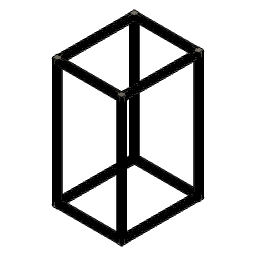
assembly (Autodesk Fusion 360 design; units mm, degrees)
Autodesk Fusion 360 part; units mm, degrees
sketch "Sketch1" plane through (0, 0, 0) normal (0, 0, 1) x (1, 0, 0) in component "2020-angle-connector"
  line L0 (10, 10) -> (-10, 10)
  line L1 (-10, 10) -> (-10, -10)
  line L2 (-10, -10) -> (10, -10)
  line L3 (10, -10) -> (10, 10)
  line L4 (10, 10) -> (-10, -10) construction
  line L5 (-10, 10) -> (10, -10) construction
  dimension "d1" = 20
  dimension "d2" = 20
  constraint horizontal L0
  constraint perpendicular L0 L1
  constraint parallel L0 L2
  constraint parallel L1 L3
  constraint coincident L4 origin
  constraint coincident L5 origin
  measures "d1" distance of L1.end L2.end
  measures "d2" distance of L0.end L1.end
extrude "Extrude1" add sketch "Sketch1" along normal blind 5 makes body 1 in component "2020-angle-connector"
fillet "Fillet1" radius 1.5 4 edges at (10, -10, 2.5) (-10, -10, 2.5) (10, 10, 2.5) (-10, 10, 2.5) on bodies 1 in component "2020-angle-connector"
sketch "Sketch2" plane through (0, -10, 0) normal (0, -1, 0) x (1, 0, 0) in component "2020-angle-connector"
  line L0 (-8.5, 5) -> (-8.5, 0)
  line L1 (-8.5, 0) -> (8.5, 0)
  line L2 (8.5, 0) -> (8.5, 5)
  line L3 (8.5, 5) -> (-8.5, 5)
  line L4 (-3, 5) -> (3, 5)
  line L5 (3, 5) -> (5, 3)
  line L6 (5, 3) -> (5, 1.5)
  line L7 (5, 1.5) -> (3, 1.5)
  line L8 (3, 1.5) -> (3, 0)
  line L9 (3, 0) -> (-3, 0)
  line L10 (-3, 0) -> (-3, 1.5)
  line L11 (-3, 1.5) -> (-5, 1.5)
  line L12 (-5, 1.5) -> (-5, 3)
  line L13 (-5, 3) -> (-3, 5)
  dimension "d7" = 10
  dimension "d8" = 6
  dimension "d9" = 135
  dimension "d11" = 1.5
  dimension "d12" = 6
  constraint parallel L3 L4
  constraint perpendicular L4 L6
  constraint perpendicular L6 L7
  constraint coincident L1 L8.end
  constraint perpendicular L1 L8
  constraint coincident L1 L9.end
  constraint perpendicular L9 L10
  constraint perpendicular L10 L11
  constraint perpendicular L11 L12
  constraint midpoint origin L9
  constraint midpoint L3 L4
  constraint equal L5 L13
  constraint equal L6 L12
  constraint equal L7 L11
  constraint equal L8 L10
  measures "d7" distance of L6 L12
  measures "d8" distance of L8 L10
  measures "d9" angle of L12 L13
  measures "d11" distance of L9.end L11
  measures "d12" distance of L4.start L4.end
extrude "Extrude2" add sketch "Sketch2" along normal blind 15.5 contours L1 L3 L4 L5 L6 L7 L8 L9 L10 L11 L12 L13 bodies 1 in component "2020-angle-connector"
pattern_circular "C-Pattern1" count 2 over 90 about axis through (0, 0, 1.75) along (0, 0, 1) of "Extrude2" in component "2020-angle-connector"
sketch "Sketch3" plane through (0, 0, 5) normal (0, 0, 1) x (-1, 0, 0) in component "2020-angle-connector"
  arc A0 (8.5, -10) -> (10, -8.5) centre (8.5, -8.5) ccw
  line L0 (10, -8.5) -> (10, 8.5)
  arc A1 (10, 8.5) -> (8.5, 10) centre (8.5, 8.5) ccw
  line L1 (8.5, 10) -> (3, 10)
  line L2 (3, 10) -> (3, 25.5)
  line L3 (3, 25.5) -> (-3, 25.5)
  line L4 (-3, 25.5) -> (-3, 10)
  line L5 (-3, 10) -> (-8.5, 10)
  arc A2 (-8.5, 10) -> (-10, 8.5) centre (-8.5, 8.5) ccw
  line L6 (-10, 8.5) -> (-10, 3)
  line L7 (-10, 3) -> (-25.5, 3)
  line L8 (-25.5, 3) -> (-25.5, -3)
  line L9 (-25.5, -3) -> (-10, -3)
  line L10 (-10, -3) -> (-10, -8.5)
  arc A3 (-10, -8.5) -> (-8.5, -10) centre (-8.5, -8.5) ccw
  line L11 (-8.5, -10) -> (8.5, -10)
  line L12 (10, -3) -> (10, 3)
  line L13 (10, 3) -> (8.5, 3)
  line L14 (8.5, 3) -> (8.5, 5)
  line L15 (8.5, 5) -> (7, 5)
  line L16 (7, 5) -> (5, 3)
  line L17 (5, 3) -> (5, -3)
  line L18 (5, -3) -> (7, -5)
  line L19 (7, -5) -> (8.5, -5)
  line L20 (8.5, -5) -> (8.5, -3)
  line L21 (8.5, -3) -> (10, -3)
  line L22 (5, 0) -> (10, 0) construction
  dimension "d17" = 6
  dimension "d18" = 10
  dimension "d19" = 1.5
  dimension "d20" = 5
  dimension "d21" = 6
  constraint coincident L0 L12.start
  constraint coincident L0 L12.end
  constraint perpendicular L0 L13
  constraint perpendicular L13 L14
  constraint perpendicular L14 L15
  constraint perpendicular L15 L17
  constraint perpendicular L16 L18
  constraint perpendicular L17 L19
  constraint perpendicular L19 L20
  constraint horizontal L21
  constraint equal L13 L21
  constraint equal L14 L20
  constraint equal L15 L19
  constraint equal L16 L18
  constraint midpoint L17 L22.start
  constraint midpoint L12 L22.end
  constraint midpoint L0 L12
  measures "d17" distance of L12.start L12.end
  measures "d18" distance of L15 L19
  measures "d19" distance of L12.start L20.end
  measures "d20" distance of L12 L17
  measures "d21" distance of L16.end L17.end
extrude "Extrude3" add sketch "Sketch3" along normal blind 15.5 contours L0 L12 L13 L14 L15 L16 L17 L18 L19 L20 L21 bodies 1 in component "2020-angle-connector"
pattern_circular "C-Pattern2" count 2 over 90 about axis through (0, 0, 1.75) along (0, 0, -1) of "Extrude3" in component "2020-angle-connector"
sketch "Sketch1 (2)" plane through (0, 0, 0) normal (0, 0, 1) x (1, 0, 0) in component "2020-profile-222,25"
  line L0 (-4.5, 0) -> (-4.5, 3.4393)
  line L1 (-7.0607, 6) -> (-8.5, 6)
  line L2 (-8.5, 6) -> (-8.5, 3)
  line L3 (-8.5, 3) -> (-10, 3)
  line L4 (-10, 3) -> (-10, 8.5)
  arc A0 (-8.5, 10) -> (-10, 8.5) centre (-8.5, 8.5) ccw
  line L5 (-8.5, 10) -> (-3, 10)
  line L6 (-3, 10) -> (-3, 8.5)
  line L7 (-3, 8.5) -> (-6, 8.5)
  line L8 (-6, 8.5) -> (-6, 7.0607)
  line L9 (-3.4393, 4.5) -> (0, 4.5)
  line L10 (0, 4.5) -> (0, 0)
  line L11 (0, 0) -> (-4.5, 0)
  line L12 (-7.0607, 6) -> (-4.5, 3.4393)
  line L13 (-6, 7.0607) -> (-3.4393, 4.5)
  circle A1 centre (0, 0) radius 2.75
  dimension "d26" = 10
  dimension "d27" = 1.5
  dimension "d28" = 4
  dimension "d29" = 5.5
  dimension "d30" = 10
  dimension "d31" = 6
  dimension "d33" = 1.5
  dimension "d34" = 3
  dimension "d35" = 5.5
  constraint vertical L0
  constraint perpendicular L0 L1
  constraint perpendicular L1 L2
  constraint perpendicular L0 L3
  constraint perpendicular L3 L4
  constraint tangent L4 A0
  constraint tangent A0 L5
  constraint perpendicular L4 L5
  constraint perpendicular L3 L6
  constraint perpendicular L6 L7
  constraint perpendicular L7 L8
  constraint perpendicular L8 L9
  constraint equal L1 L8
  constraint equal L2 L7
  constraint equal L3 L6
  constraint equal L4 L5
  constraint equal L0 L9
  constraint coincident L10.end L11.start
  constraint perpendicular L9 L10
  constraint horizontal L11
  constraint parallel L12 L13
  constraint equal L10 L11
  measures "d26" distance of L4 L10
  measures "d27" radius of A0
  measures "d28" distance of L0 L2
  measures "d29" distance of L0 L4
  measures "d30" distance of L10.end L5
  measures "d31" distance of L1 L11
  measures "d33" distance of L12 L13
  measures "d34" distance of L3 L11
  measures "d35" diameter of A1
extrude "Extrude1'" add sketch "Sketch1 (2)" along normal mid plane 222.25 separate body contours L0 L1 L2 L3 L4 A0 L5 L6 L7 L8 L9 L10 L11 L12 L13 A1 makes body 2 in component "2020-profile-222,25"
fillet "Fillet1'" radius 0.5 3 edges at (-8.5, 6, 0) (-7.0607, 6, 0) (-4.5, 3.4393, 0) on bodies 2 in component "2020-profile-222,25"
fillet "Fillet2" radius 0.25 4 edges at (-8.5, 3, 0) (-10, 3, 0) (-3, 10, 0) (-3, 8.5, 0) on bodies 2 in component "2020-profile-222,25"
fillet "Fillet3" radius 0.5 2 edges at (-6, 7.0607, 0) (-3.4393, 4.5, 0) on bodies 2 in component "2020-profile-222,25"
mirror "Mirror1" about plane through (0, 0, 0) normal (1, 0, 0) of bodies 2 merged in component "2020-profile-222,25"
mirror "Mirror2" about plane through (0, 0, 0) normal (0, 1, 0) of bodies 2 merged in component "2020-profile-222,25"
sketch "Sketch1 (3)" plane through (0, 0, 0) normal (0, 0, 1) x (1, 0, 0) in component "2020-profile-476"
  line L0 (-4.5, 0) -> (-4.5, 3.4393)
  line L1 (-7.0607, 6) -> (-8.5, 6)
  line L2 (-8.5, 6) -> (-8.5, 3)
  line L3 (-8.5, 3) -> (-10, 3)
  line L4 (-10, 3) -> (-10, 8.5)
  arc A0 (-8.5, 10) -> (-10, 8.5) centre (-8.5, 8.5) ccw
  line L5 (-8.5, 10) -> (-3, 10)
  line L6 (-3, 10) -> (-3, 8.5)
  line L7 (-3, 8.5) -> (-6, 8.5)
  line L8 (-6, 8.5) -> (-6, 7.0607)
  line L9 (-3.4393, 4.5) -> (0, 4.5)
  line L10 (0, 4.5) -> (0, 0)
  line L11 (0, 0) -> (-4.5, 0)
  line L12 (-7.0607, 6) -> (-4.5, 3.4393)
  line L13 (-6, 7.0607) -> (-3.4393, 4.5)
  circle A1 centre (0, 0) radius 2.75
  dimension "d26_1" = 10
  dimension "d27_1" = 1.5
  dimension "d28_1" = 4
  dimension "d29_1" = 5.5
  dimension "d30_1" = 10
  dimension "d31_1" = 6
  dimension "d33_1" = 1.5
  dimension "d34_1" = 3
  dimension "d35_1" = 5.5
  constraint vertical L0
  constraint perpendicular L0 L1
  constraint perpendicular L1 L2
  constraint perpendicular L0 L3
  constraint perpendicular L3 L4
  constraint tangent L4 A0
  constraint tangent A0 L5
  constraint perpendicular L4 L5
  constraint perpendicular L3 L6
  constraint perpendicular L6 L7
  constraint perpendicular L7 L8
  constraint perpendicular L8 L9
  constraint equal L1 L8
  constraint equal L2 L7
  constraint equal L3 L6
  constraint equal L4 L5
  constraint equal L0 L9
  constraint coincident L10.end L11.start
  constraint perpendicular L9 L10
  constraint horizontal L11
  constraint parallel L12 L13
  constraint equal L10 L11
  measures "d26_1" distance of L4 L10
  measures "d27_1" radius of A0
  measures "d28_1" distance of L0 L2
  measures "d29_1" distance of L0 L4
  measures "d30_1" distance of L10.end L5
  measures "d31_1" distance of L1 L11
  measures "d33_1" distance of L12 L13
  measures "d34_1" distance of L3 L11
  measures "d35_1" diameter of A1
extrude "Extrude1''" add sketch "Sketch1 (3)" along normal blind 476 separate body contours L0 L1 L2 L3 L4 A0 L5 L6 L7 L8 L9 L10 L11 L12 L13 A1 makes body 3 in component "2020-profile-476"
fillet "Fillet1''" radius 0.5 3 edges at (-8.5, 6, 238) (-7.0607, 6, 238) (-4.5, 3.4393, 238) on bodies 3 in component "2020-profile-476"
fillet "Fillet2'" radius 0.25 4 edges at (-8.5, 3, 238) (-10, 3, 238) (-3, 10, 238) (-3, 8.5, 238) on bodies 3 in component "2020-profile-476"
fillet "Fillet3'" radius 0.5 2 edges at (-6, 7.0607, 238) (-3.4393, 4.5, 238) on bodies 3 in component "2020-profile-476"
mirror "Mirror1'" about plane through (0, 0, 0) normal (1, 0, 0) of bodies 3 merged in component "2020-profile-476"
mirror "Mirror2'" about plane through (0, 0, 0) normal (0, 1, 0) of bodies 3 merged in component "2020-profile-476"
sketch "Sketch1 (4)" plane through (0, 0, 0) normal (0, 0, 1) x (1, 0, 0) in component "2020-profile-270"
  line L0 (-4.5, 0) -> (-4.5, 3.4393)
  line L1 (-7.0607, 6) -> (-8.5, 6)
  line L2 (-8.5, 6) -> (-8.5, 3)
  line L3 (-8.5, 3) -> (-10, 3)
  line L4 (-10, 3) -> (-10, 8.5)
  arc A0 (-8.5, 10) -> (-10, 8.5) centre (-8.5, 8.5) ccw
  line L5 (-8.5, 10) -> (-3, 10)
  line L6 (-3, 10) -> (-3, 8.5)
  line L7 (-3, 8.5) -> (-6, 8.5)
  line L8 (-6, 8.5) -> (-6, 7.0607)
  line L9 (-3.4393, 4.5) -> (0, 4.5)
  line L10 (0, 4.5) -> (0, 0)
  line L11 (0, 0) -> (-4.5, 0)
  line L12 (-7.0607, 6) -> (-4.5, 3.4393)
  line L13 (-6, 7.0607) -> (-3.4393, 4.5)
  circle A1 centre (0, 0) radius 2.75
  dimension "d26_2" = 10
  dimension "d27_2" = 1.5
  dimension "d28_2" = 4
  dimension "d29_2" = 5.5
  dimension "d30_2" = 10
  dimension "d31_2" = 6
  dimension "d33_2" = 1.5
  dimension "d34_2" = 3
  dimension "d35_2" = 5.5
  constraint vertical L0
  constraint perpendicular L0 L1
  constraint perpendicular L1 L2
  constraint perpendicular L0 L3
  constraint perpendicular L3 L4
  constraint tangent L4 A0
  constraint tangent A0 L5
  constraint perpendicular L4 L5
  constraint perpendicular L3 L6
  constraint perpendicular L6 L7
  constraint perpendicular L7 L8
  constraint perpendicular L8 L9
  constraint equal L1 L8
  constraint equal L2 L7
  constraint equal L3 L6
  constraint equal L4 L5
  constraint equal L0 L9
  constraint coincident L10.end L11.start
  constraint perpendicular L9 L10
  constraint horizontal L11
  constraint parallel L12 L13
  constraint equal L10 L11
  measures "d26_2" distance of L4 L10
  measures "d27_2" radius of A0
  measures "d28_2" distance of L0 L2
  measures "d29_2" distance of L0 L4
  measures "d30_2" distance of L10.end L5
  measures "d31_2" distance of L1 L11
  measures "d33_2" distance of L12 L13
  measures "d34_2" distance of L3 L11
  measures "d35_2" diameter of A1
extrude "Extrude1'''" add sketch "Sketch1 (4)" along normal blind 270 separate body contours L0 L1 L2 L3 L4 A0 L5 L6 L7 L8 L9 L10 L11 L12 L13 A1 makes body 4 in component "2020-profile-270"
fillet "Fillet1'''" radius 0.5 3 edges at (-8.5, 6, 135) (-7.0607, 6, 135) (-4.5, 3.4393, 135) on bodies 4 in component "2020-profile-270"
fillet "Fillet2''" radius 0.25 4 edges at (-8.5, 3, 135) (-10, 3, 135) (-3, 10, 135) (-3, 8.5, 135) on bodies 4 in component "2020-profile-270"
fillet "Fillet3''" radius 0.5 2 edges at (-6, 7.0607, 135) (-3.4393, 4.5, 135) on bodies 4 in component "2020-profile-270"
mirror "Mirror1''" about plane through (0, 0, 0) normal (1, 0, 0) of bodies 4 merged in component "2020-profile-270"
mirror "Mirror2''" about plane through (0, 0, 0) normal (0, 1, 0) of bodies 4 merged in component "2020-profile-270"
component "2020-profile-222,25" placed x (0, 0, -1) y (0, 1, 0) z (1, 0, 0) at (0, -145, 10)
component "2020-angle-connector" placed x (-1, 0, 0) y (0, -1, 0) z (0, 0, 1) at (121.125, -145, 0)
component "2020-profile-476" placed x (1, 0, 0) y (0, 1, 0) z (0, 0, 1) at (121.125, -145, 5)
component "2020-profile-270" placed x (1, 0, 0) y (0, 0, -1) z (0, 1, 0) at (121.125, -135, 10)
component "2020-angle-connector" placed x (0, 1, 0) y (-1, 0, 0) z (0, 0, 1) at (-121.125, -145, 0)
component "2020-profile-270" placed x (1, 0, 0) y (0, 0, -1) z (0, 1, 0) at (-121.125, -135, 10)
component "2020-profile-476" placed x (1, 0, 0) y (0, 1, 0) z (0, 0, 1) at (-121.125, -145, 5)
component "2020-angle-connector" placed x (0, -1, 0) y (1, 0, 0) z (0, 0, 1) at (121.125, 145, 0)
component "2020-angle-connector" placed x (1, 0, 0) y (0, 1, 0) z (0, 0, 1) at (-121.125, 145, 0)
component "2020-angle-connector" placed x (0, 1, 0) y (1, 0, 0) z (0, 0, -1) at (121.125, -145, 486)
component "2020-profile-222,25" placed x (0, 0, -1) y (0, -1, 0) z (-1, 0, 0) at (0, 145, 10)
component "2020-profile-476" placed x (0, 1, 0) y (-1, 0, 0) z (0, 0, 1) at (121.125, 145, 5)
component "2020-profile-476" placed x (0, -1, 0) y (1, 0, 0) z (0, 0, 1) at (-121.125, 145, 5)
component "2020-angle-connector" placed x (1, 0, 0) y (0, -1, 0) z (0, 0, -1) at (-121.125, -145, 486)
component "2020-angle-connector" placed x (0, -1, 0) y (-1, 0, 0) z (0, 0, -1) at (-121.125, 145, 486)
component "2020-angle-connector" placed x (-1, 0, 0) y (0, 1, 0) z (0, 0, -1) at (121.125, 145, 486)
component "2020-profile-270" placed x (1, 0, 0) y (0, 0, 1) z (0, -1, 0) at (121.125, 135, 476)
component "2020-profile-270" placed x (1, 0, 0) y (0, 0, 1) z (0, -1, 0) at (-121.125, 135, 476)
component "2020-profile-222,25" placed x (0, 0, 1) y (0, -1, 0) z (1, 0, 0) at (0, -145, 476)
component "2020-profile-222,25" placed x (0, 0, 1) y (0, -1, 0) z (1, 0, 0) at (0, 145, 476)
